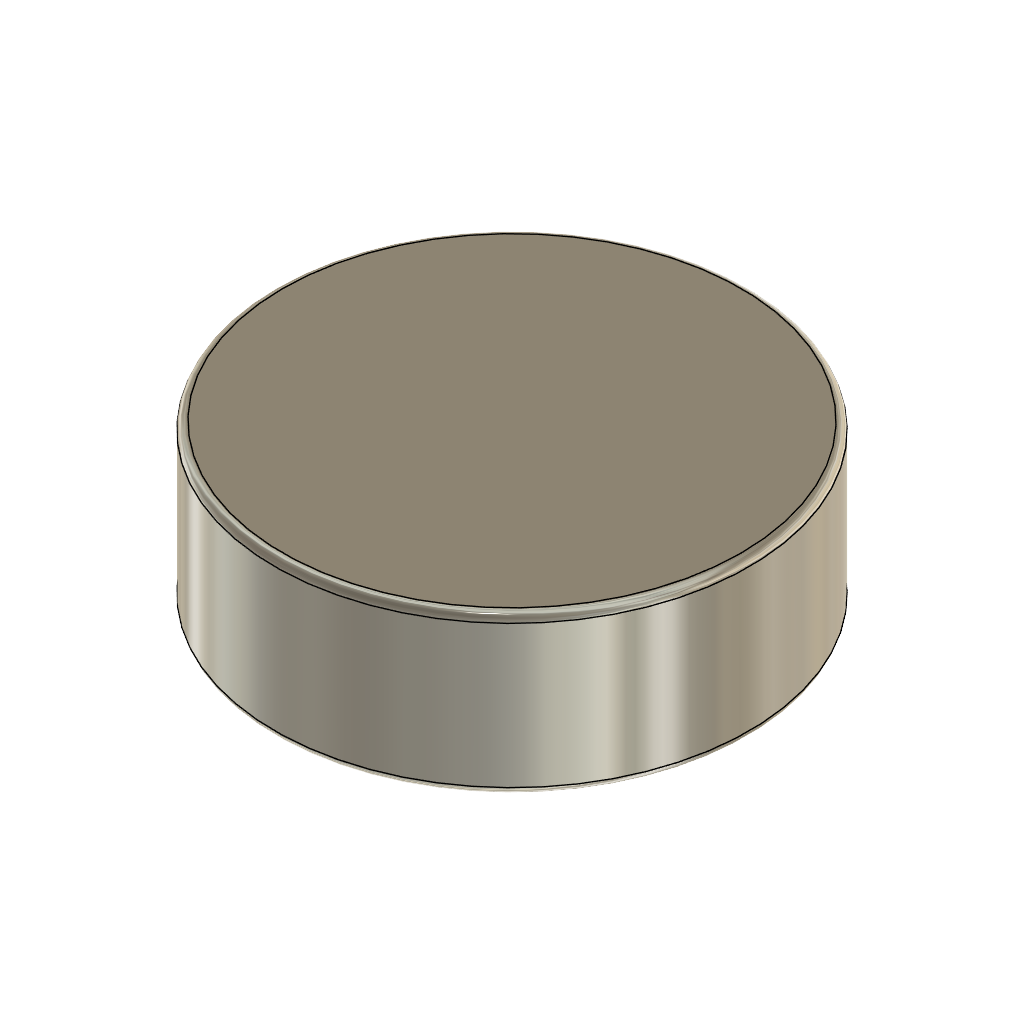
3_mm_x_1_mm_neodymium_disc_magnet (Autodesk Fusion 360 design; units mm, degrees)
Autodesk Fusion 360 part; units mm, degrees
sketch "3 mm x 1 mm neodymium disc magnet" plane through (0, 0, 0) normal (0, 0, 1) x (1, 0, 0)
  circle A0 centre (0, 0) radius 1.5
  dimension "d1" = 3
  constraint coincident A0.centre origin
  measures "d1" diameter of A0
extrude "Extrude1" add sketch "3 mm x 1 mm neodymium disc magnet" along normal blind 1
fillet "Fillet1" radius 0.05 2 edges at (-1.3985, -0.5424, 1) (-1.3985, -0.5424, 0)
named bodies: "3 mm x 1 mm Neodymium Disc Magnet"
